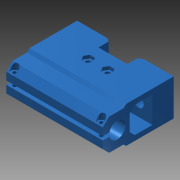
# Autodesk Inventor part: XCarriage
Saved by Autodesk Inventor 2015 (Build 190159000, 159)
## iProperties
Created: 2014-08-15
Part Number: XCarriage
Material: ABS Plastic
Document SubType Name: Modeling
Designer: t_clevj
Density: 1.06 g/cm^3
Appearance: Cyan
Author: t_clevj
Autodesk Inventor part; units mm, degrees
ref_plane "YZ Plane" through (0, 0, 0) normal (1, 0, 0) x (0, 1, 0)
ref_plane "XZ Plane" through (0, 0, 0) normal (0, 1, 0) x (-1, 0, 0)
ref_plane "XY Plane" through (0, 0, 0) normal (0, 0, 1) x (1, 0, 0)
sketch "Sketch1" plane through (0, 0, 0) normal (1, 0, 0) x (0, 1, 0)
  arc A0 (-6.3246, -1.5) -> (-6.3246, 1.5) centre (0, 0) ccw
  line L0 (-11.5, 1.5) -> (-11.5, 12.5)
  line L1 (-11.5, 12.5) -> (35, 12.5)
  line L2 (-11.5, -1.5) -> (-11.5, -12.5)
  line L3 (-11.5, -12.5) -> (35, -12.5)
  line L4 (-11.5, 1.5) -> (-6.3246, 1.5)
  line L5 (-11.5, -1.5) -> (-6.3246, -1.5)
  line L6 (35, 12.5) -> (35, -12.5)
  dimension "d0" = 13
  dimension "d1" = 1.5
  dimension "d2" = 1.5
  dimension "d3" = 11.5
  dimension "d4" = 12.5
  dimension "d5" = 12.5
  dimension "d140" = 35
  constraints: 14 end point, 3 vertical, 2 horizontal, 2 point on circle, 2 vertical alignment, 1 centre point, 1 coincident, 1 parallel, 1 perpendicular
  measures "d0" diameter of A0
  measures "d1" vertical distance of point (0, 0) L2.start
  measures "d2" vertical distance of point (0, 0) L0.start
  measures "d3" distance from line of point (0, 0) L0
  measures "d4" distance from line of point (0, 0) L1
  measures "d5" distance from line of L3 point (0, 0)
  measures "d140" distance from line of L6 point (0, 0)
extrude "MainBlock" add sketch "Sketch1" along normal blind 77
chamfer "BearingHolderChamfer" distance 5 angle 45 2 edges at (38.5, -11.5, 12.5) (38.5, -11.5, -12.5)
sketch "Sketch2" plane through (0, 35, 12.5) normal (0, 0, 1) x (1, 0, 0)
  line L0 (77, -46.5) -> (77, -41.5) projected
  line L1 (77, -41.5) -> (0, -41.5) projected
  line L2 (0, -41.5) -> (0, -46.5) projected
  line L3 (0, -46.5) -> (77, -46.5) projected
  point P0 (0, -35)
  point P1 (4, -43.75)
  point P2 (73, -43.75)
  dimension "d17" = 2.75
  dimension "d18" = 4
  dimension "d19" = 4
  constraints: 1 horizontal alignment
  measures "d17" distance from line of L3 point (73, -43.75)
  measures "d18" distance from line of L0 point (73, -43.75)
  measures "d19" distance from line of L2 point (4, -43.75)
hole "BearingHolderClamp" at (4, -8.75, 12.5) at (73, -8.75, 12.5) direction (0, 0, -1) diameter 3 depth 25 tip angle 118 counterbore diameter 5.5 counterbore depth 5
sketch "Sketch3" plane through (77, 35, -12.5) normal (0, 0, -1) x (-1, 0, 0)
  circle A0 centre (73, -43.75) radius 1.5 projected
  circle A1 centre (73, -43.75) radius 1.5 projected
  circle A2 centre (4, -43.75) radius 1.5 projected
  circle A3 centre (4, -43.75) radius 1.5 projected
  line L0 (7.1754, -43.75) -> (5.5877, -46.5)
  line L1 (5.5877, -46.5) -> (2.4123, -46.5)
  line L2 (2.4123, -46.5) -> (0.8246, -43.75)
  line L3 (0.8246, -43.75) -> (2.4123, -41)
  line L4 (2.4123, -41) -> (5.5877, -41)
  line L5 (5.5877, -41) -> (7.1754, -43.75)
  line L6 (76.1754, -43.75) -> (74.5877, -46.5)
  line L7 (74.5877, -46.5) -> (71.4123, -46.5)
  line L8 (71.4123, -46.5) -> (69.8246, -43.75)
  line L9 (69.8246, -43.75) -> (71.4123, -41)
  line L10 (71.4123, -41) -> (74.5877, -41)
  line L11 (74.5877, -41) -> (76.1754, -43.75)
  point P0 (77, -35)
  dimension "d27" = 5.5
  dimension "d28" = 5.5
  constraints: 24 end point, 2 coincident, 2 horizontal, 26 other
  measures "d27" distance between parallel lines of L1 L4
  measures "d28" distance between parallel lines of L7 L10
extrude "BearingHolderNutTrap" cut sketch "Sketch3" against normal blind 5
sketch "Sketch4" plane through (0, 0, 0) normal (-1, 0, 0) x (0, 0, 1)
  arc A0 (1.5, -6.3246) -> (-1.5, -6.3246) centre (0, 0) ccw projected
  line L0 (-12.5, 35) -> (-12.5, -6.5) projected
  line L1 (10.5, 10) -> (-10.5, 10)
  line L2 (-10.5, 10) -> (-10.5, 28)
  line L3 (-10.5, 28) -> (10.5, 28)
  line L4 (10.5, 28) -> (10.5, 10)
  dimension "d31" = 18
  dimension "d32" = 21
  dimension "d33" = 10
  dimension "d34" = 2
  constraints: 8 end point, 2 parallel, 1 horizontal, 1 perpendicular
  measures "d31" distance of L1.end L2.end
  measures "d32" distance of L1.start L1.end
  measures "d33" distance from line of A0.centre L1
  measures "d34" distance between parallel lines of L0 L2
extrude "BeltCutoutY" cut sketch "Sketch4" against normal up to surface (77 mm away)
sketch "Sketch5" plane through (0, 35, 12.5) normal (0, 1, 0) x (1, 0, 0)
  line L0 (77, 25) -> (77, 0) projected
  line L1 (0, 25) -> (77, 25) projected
  line L2 (27, 2) -> (50, 2)
  line L3 (50, 2) -> (50, 23)
  line L4 (50, 23) -> (27, 23)
  line L5 (27, 23) -> (27, 2)
  point P0 (0, 12.5)
  dimension "d37" = 21
  dimension "d38" = 23
  dimension "d39" = 2
  dimension "d40" = 27
  constraints: 8 end point, 2 parallel, 1 horizontal, 1 perpendicular
  measures "d37" distance of L4.end L2.start
  measures "d38" distance of L2.start L2.end
  measures "d39" distance between parallel lines of L1 L4
  measures "d40" distance between parallel lines of L0 L3
extrude "BeltCutoutX" cut sketch "Sketch5" against normal up to surface (7 mm away)
sketch "Sketch6" plane through (77, 35, -12.5) normal (0, 0, -1) x (-1, 0, 0)
  line L0 (77, 0) -> (77, -41.5) projected
  line L1 (77, 0) -> (0, 0) projected
  line L2 (0, -41.5) -> (0, 0) projected
  line L3 (0, -28) -> (77, -28)
  point P0 (77, -35)
  dimension "d43" = 28
  constraints: 2 end point, 2 point on line, 1 perpendicular
  measures "d43" distance between parallel lines of L1 L3
extrude "BoltPadUpper" add sketch "Sketch6" along normal blind 2
sketch "Sketch7" plane through (0, 35, 12.5) normal (0, 0, 1) x (1, 0, 0)
  line L0 (77, 0) -> (77, -41.5) projected
  line L1 (0, 0) -> (77, 0) projected
  line L2 (0, -41.5) -> (0, 0) projected
  line L3 (0, -28) -> (0, 0) projected
  line L4 (0, -28) -> (77, -28)
  line L5 (77, 0) -> (77, -28) projected
  point P0 (0, -35)
  dimension "d46" = 28
  constraints: 2 end point, 2 point on line, 1 perpendicular
  measures "d46" distance between parallel lines of L1 L4
extrude "BoltPadLower" add sketch "Sketch7" along normal blind 2
chamfer "BoltPadChamfer" distance 2 angle 45 2 edges at (38.5, 7, 12.5) (38.5, 7, -12.5)
sketch "Sketch8" plane through (77, 35, -14.5) normal (0, 0, -1) x (-1, 0, 0)
  line L0 (77, 0) -> (0, 0) projected
  line L1 (0, 0) -> (0, -28) projected
  point P0 (77, -35)
  point P1 (30.75, -12)
  point P2 (46.25, -12)
  dimension "d54" = 12
  dimension "d116" = 15.5
  dimension "d117" = 30.75
  constraints: 1 horizontal alignment
  measures "d54" distance from line of L0 point (46.25, -12)
  measures "d116" distance of point (46.25, -12) point (30.75, -12)
  measures "d117" distance from line of L1 point (30.75, -12)
hole "BearingBoltHoles" at (46.25, 23, -14.5) at (30.75, 23, -14.5) direction (0, 0, 1) diameter 4 end up to face face through (25.6667, 25.6667, 14.5) facing (0, 0, 1) counterbore diameter 7 counterbore depth 1.5
chamfer "BearingCutoutYChamfer" distance 4 angle 45 2 edges at (38.5, 10, 10.5) (38.5, 10, -10.5)
sketch "Sketch9" plane through (50, 35, 10.5) normal (0, 0, -1) x (-1, 0, 0)
  line L0 (50, -7) -> (23, -7) projected
  line L1 (23, 0) -> (23, -7) projected
  line L2 (0, 0) -> (0, -7) projected
  line L3 (0, -7) -> (-27, -7) projected
  circle A0 centre (19.25, -12) radius 2 projected
  circle A1 centre (3.75, -12) radius 2 projected
  arc A2 (0, -1.6589) -> (-6.048, -7) centre (3.75, -12) ccw
  arc A3 (29.048, -7) -> (23, -1.6589) centre (19.25, -12) ccw
  line L4 (0, -1.6589) -> (0, -7)
  line L5 (0, -7) -> (-6.048, -7)
  line L6 (23, -1.6589) -> (23, -7)
  line L7 (23, -7) -> (29.048, -7)
  point P0 (50, -35)
  dimension "d67" = 11
  dimension "d68" = 11
  constraints: 8 end point, 4 collinear, 4 point on circle, 4 point on line, 2 centre point, 2 coincident
  measures "d67" radius of A3
  measures "d68" radius of A2
sketch "Sketch10" plane through (0, 35, 14.5) normal (0, 0, 1) x (1, 0, 0)
  circle A0 centre (46.25, -12) radius 2 projected
  circle A1 centre (30.75, -12) radius 2 projected
  line L0 (34.7915, -12) -> (32.7707, -15.5)
  line L1 (32.7707, -15.5) -> (28.7293, -15.5)
  line L2 (28.7293, -15.5) -> (26.7085, -12)
  line L3 (26.7085, -12) -> (28.7293, -8.5)
  line L4 (28.7293, -8.5) -> (32.7707, -8.5)
  line L5 (32.7707, -8.5) -> (34.7915, -12)
  line L6 (50.2915, -12) -> (48.2707, -15.5)
  line L7 (48.2707, -15.5) -> (44.2293, -15.5)
  line L8 (44.2293, -15.5) -> (42.2085, -12)
  line L9 (42.2085, -12) -> (44.2293, -8.5)
  line L10 (44.2293, -8.5) -> (48.2707, -8.5)
  line L11 (48.2707, -8.5) -> (50.2915, -12)
  point P0 (0, -35)
  dimension "d71" = 7
  constraints: 24 end point, 2 coincident, 2 horizontal, 1 collinear, 26 other
  measures "d71" distance between parallel lines of L1 L4
extrude "BearingNutTrap" cut sketch "Sketch10" against normal blind 2.5
sketch "Sketch11" plane through (77, 35, -14.5) normal (0, 0, -1) x (-1, 0, 0)
  line L0 (77, 0) -> (0, 0) projected
  line L1 (0, 10) -> (24, 10)
  line L2 (77, 10) -> (53, 10)
  line L3 (77, 10) -> (77, 0)
  line L4 (0, 0) -> (0, 10)
  line L5 (27, 0) -> (27, 0)
  line L6 (50, 0) -> (50, 0)
  line L7 (27, 0) -> (27, 8)
  line L8 (27, 0) -> (27, -7) projected
  line L9 (50, 0) -> (50, 8)
  line L10 (53, 10) -> (50, 8)
  line L11 (24, 10) -> (27, 8)
  point P0 (77, -35)
  point P1 (26, -4.2326)
  dimension "d74" = 24
  dimension "d75" = 24
  dimension "d80" = 10
  dimension "d93" = 8
  constraints: 20 end point, 3 vertical, 2 horizontal, 2 perpendicular, 1 horizontal alignment, 1 parallel, 1 point on line, 1 other
  measures "d74" distance of L1.start L1.end
  measures "d75" distance of L2.start L2.end
  measures "d80" distance of L2.start L0.start
  measures "d93" distance of L5.end L7.end
extrude "XRodHolderPad" add sketch "Sketch11" against normal up to surface (29 mm away)
sketch "Sketch15" plane through (0, 45, -14.5) normal (0, 1, 0) x (1, 0, 0)
  line L0 (53, -29) -> (77, -29) projected
  line L1 (77, 0) -> (77, -29) projected
  line L2 (53, 0) -> (77, 0) projected
  line L3 (53, 0) -> (53, -29) projected
  circle A0 centre (11, -14.5) radius 4
  circle A1 centre (66, -14.5) radius 4
  point P0 (0, -14.5)
  dimension "d94" = 8
  dimension "d95" = 8
  dimension "d99" = 14.5
  dimension "d136" = 55
  dimension "d137" = 11
  constraints: 2 centre point, 1 horizontal alignment
  measures "d94" diameter of A0
  measures "d95" diameter of A1
  measures "d99" distance from line of L0 A1.centre
  measures "d136" distance of A0.centre A1.centre
  measures "d137" distance from line of L1 A1.centre
extrude "XRodHole" cut sketch "Sketch15" against normal up to surface (17 mm away) contours A0 | A1
sketch "Sketch20" plane through (77, 35, -14.5) normal (0, 0, -1) x (-1, 0, 0)
  line L0 (24, 10) -> (0, 10) projected
  line L1 (0, 10) -> (0, -28) projected
  line L2 (77, -28) -> (77, 10) projected
  point P0 (77, -35)
  point P1 (66, 2)
  point P2 (11, 2)
  dimension "d122" = 8
  dimension "d123" = 11
  dimension "d124" = 11
  constraints: 1 horizontal alignment
  measures "d122" distance from line of L0 point (11, 2)
  measures "d123" distance from line of L1 point (11, 2)
  measures "d124" distance from line of L2 point (66, 2)
hole "Hole3" at (11, 37, -14.5) at (66, 37, -14.5) direction (0, 0, 1) diameter 3 depth 10 counterbore diameter 5.5 counterbore depth 3.7
ref_plane "Work Plane3" through (0, 35, -1) normal (0, 0, 1) x (1, 0, 0)
sketch "Sketch21" plane through (0, 35, -1) normal (0, 0, 1) x (1, 0, 0)
  circle A0 centre (11, 2) radius 1.5 projected
  circle A1 centre (66, 2) radius 1.5 projected
  line L0 (11, 5.1754) -> (13.75, 3.5877)
  line L1 (13.75, 3.5877) -> (13.75, 0.4123)
  line L2 (13.75, 0.4123) -> (11, -1.1754)
  line L3 (11, -1.1754) -> (8.25, 0.4123)
  line L4 (8.25, 0.4123) -> (8.25, 3.5877)
  line L5 (8.25, 3.5877) -> (11, 5.1754)
  line L6 (66, 5.1754) -> (68.75, 3.5877)
  line L7 (68.75, 3.5877) -> (68.75, 0.4123)
  line L8 (68.75, 0.4123) -> (66, -1.1754)
  line L9 (66, -1.1754) -> (63.25, 0.4123)
  line L10 (63.25, 0.4123) -> (63.25, 3.5877)
  line L11 (63.25, 3.5877) -> (66, 5.1754)
  point P0 (0, -35)
  dimension "d133" = 5.5
  constraints: 24 end point, 2 coincident, 2 vertical, 1 parallel, 26 other
  measures "d133" distance between parallel lines of L7 L10
extrude "Extrusion18" cut sketch "Sketch21" against normal blind 6.8
extrude "Extrusion19" cut sketch "Sketch9" along normal up to surface (21 mm away) contours L0 L1 A3 | L2 L3 A2
sketch "Sketch26" plane through (50, 35, 10.5) normal (0, 0, -1) x (-1, 0, 0)
  circle A0 centre (3.75, -12) radius 2 projected
  circle A1 centre (3.75, -12) radius 4.75
  point P0 (50, -35)
  dimension "d151" = 9.5
  constraints: 1 centre point, 1 coincident
  measures "d151" diameter of A1
extrude "Extrusion24" cut sketch "Sketch26" against normal blind 0.25
body "Solid1"
